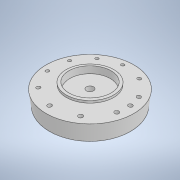
# Autodesk Inventor part: top
Saved by Autodesk Inventor 2022 (Build 260153000, 153)
## iProperties
Created: 2022-06-04
Part Number: top
Material: Generic
Document SubType Name: Modeling
Designer: Jacob
Density: 1 g/cm^3
Appearance: Default
Author: Jacob
Autodesk Inventor part; units mm, degrees
ref_plane "YZ Plane" through (0, 0, 0) normal (1, 0, 0) x (0, 1, 0)
ref_plane "XZ Plane" through (0, 0, 0) normal (0, 1, 0) x (-1, 0, 0)
ref_plane "XY Plane" through (0, 0, 0) normal (0, 0, 1) x (1, 0, 0)
sketch "Sketch3" plane through (0, 0, 0) normal (0, 1, 0) x (-1, 0, 0)
  circle A0 centre (0, 0) radius 16.245
  circle A1 centre (0, -25.3377) radius 1.27
  circle A2 centre (-24.0976, -7.8298) radius 1.27
  circle A3 centre (-14.8931, 20.4986) radius 1.27
  circle A4 centre (24.0976, -7.8298) radius 1.27
  circle A5 centre (24.0976, 7.8298) radius 1.27
  circle A6 centre (-24.0976, 7.8298) radius 1.27
  circle A7 centre (-14.8931, -20.4986) radius 1.27
  circle A8 centre (0, 25.3377) radius 1.27
  circle A9 centre (14.8931, -20.4986) radius 1.27
  circle A10 centre (14.8931, 20.4986) radius 1.27
  circle A11 centre (-25.3377, 0) radius 1.27
  circle A12 centre (0, 0) radius 30
  circle A13 centre (0, 0) radius 16.245
  circle A14 centre (0, 0) radius 14.245
  constraints: 15 centre point, 32 other
extrude "Extrusion4" add sketch "Sketch3" against normal blind 10 contours A0 | A12 | A14
extrude "Extrusion5" add sketch "Sketch3" along normal blind 1.5 contours A0
sketch "Sketch4" plane through (0, 1.5, 0) normal (0, 1, 0) x (1, 0, 0)
  circle A0 centre (0, 0) radius 14.245 projected
  circle A1 centre (0, 0) radius 14.345
  dimension "d16" = 0.1
  constraints: 1 centre point
  measures "d16" radial gap between concentric circles of A0 A1
extrude "Extrusion7" cut sketch "Sketch4" against normal blind 5 contours A0 | A1
sketch "Sketch5" plane through (0, -3.5, 0) normal (0, 1, 0) x (1, 0, 0)
  circle A0 centre (0, 0) radius 2.55
  dimension "d19" = 5.1
  constraints: 1 centre point, 1 coincident
  measures "d19" diameter of A0
extrude "Extrusion8" cut sketch "Sketch5" against normal up to surface (6.5 mm away)
body "Solid2"
